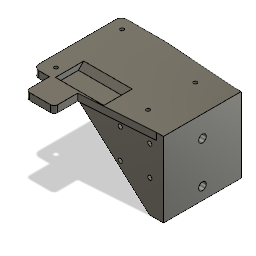
RPLIDAR Bracket v5 (Autodesk Fusion 360 design; units mm, degrees)
Autodesk Fusion 360 part; units mm, degrees
note: some values were not read from the file. Set by a fixed rule: which sketch regions a step uses.
sketch "Sketch1" plane through (0, 0, 0) normal (0, 1, 0) x (1, 0, 0)
  line L0 (0, 0) -> (-5, 0) construction
  line L1 (-5, 0) -> (-33.0162, 0) construction
  line L2 (0, 0) -> (0, 35) construction
  circle A0 centre (-28, 28) radius 1.5
  circle A1 centre (42, 20) radius 1.5
  circle A2 centre (-28, -28) radius 1.5
  circle A3 centre (42, -20) radius 1.5
  line L3 (-38, 0) -> (-38, 37.5)
  line L4 (-38, 37.5) -> (0, 37.5)
  line L5 (0, 37.5) -> (62, 33)
  line L6 (62, 33) -> (62, 0)
  line L7 (62, -33) -> (62, 0)
  line L8 (0, -37.5) -> (62, -33)
  line L9 (-38, -37.5) -> (0, -37.5)
  line L10 (-38, 0) -> (-38, -37.5)
  dimension "d1" = 3
  dimension "d2" = 3
  dimension "d3" = 40
  dimension "d4" = 56
  dimension "d5" = 70
  dimension "d6" = 42
  dimension "d7" = 75
  dimension "d8" = 100
  dimension "d9" = 10
  dimension "d10" = 33
  constraint coincident L0.start L2.start
  constraint horizontal L0
  constraint parallel L0 L1
  constraint perpendicular L0 L2
  constraint symmetric L1 A0 A2
  constraint symmetric L1 A1 A3
  constraint perpendicular L2 L4
  constraint parallel L2 L6
  constraint symmetric L1 L3.start L10.start
  constraint symmetric L1 L3.end L9.start
  constraint symmetric L1 L4.end L8.start
  constraint symmetric L1 L5.end L7.start
  constraint symmetric L1 L6.end L7.end
  constraint vertical L3
  constraint coincident L2 L4.end
  constraint coincident L6.end L7.end
  constraint coincident L3.start L10.start
  measures "d1" diameter of A0
  measures "d2" diameter of A1
  measures "d3" distance of A1.centre A3.centre
  measures "d4" distance of A0.centre A2.centre
  measures "d5" horizontal distance of A0.centre A1.centre
  measures "d6" horizontal distance of L0.start A1.centre
  measures "d7" distance of L3.end L9.start
  measures "d8" distance of L3 L6
  measures "d9" distance of A0.centre L3
  measures "d10" distance of L5.end L6.end
  measures "d20" angle of L4.end
extrude "Extrude1" add sketch "Sketch1" along normal blind 6
ref_plane "WorkPlane1" through (0, 0, 27) normal (0, 0, 1) x (1, 0, 0)
sketch "Sketch3" plane through (0, 0, 27) normal (0, 0, 1) x (1, 0, 0)
  line L0 (-8, 0) -> (62, 0)
  line L1 (62, -57.6259) -> (56, -57.6259)
  line L2 (56, -57.6259) -> (-8, 0)
  line L3 (62, 0) -> (62, -57.6259)
  line L4 (54.1896, -11.7055) -> (54.187, -11.7094)
  point P0 (5, 0)
  dimension "d19" = 6
  dimension "d20" = 42
  dimension "d21" = 70
  constraint vertical L3
  constraint perpendicular L0 L3
  constraint coincident L0.end L4
  constraint perpendicular L1 L3
  constraint coincident P0 L0
  constraint coincident origin L0
  measures "d19" distance of L1.end L1.start
  measures "d20" angle of L0 L2
  measures "d21" distance of L0.start L0.end
extrude "Extrude3" add sketch "Sketch3" along normal blind 6
mirror "Mirror1" about plane through (0, 0, 0) normal (0, 0, 1) of "Extrude3"
sketch "Sketch4" plane through (62, 0, 0) normal (1, 0, 0) x (0, 0, -1)
  line L0 (-27, 0) -> (27, 0)
  line L1 (27, 0) -> (27, -57.6259)
  line L2 (27, -57.6259) -> (33, -57.6259)
  line L3 (33, -57.6259) -> (33, 0)
  line L4 (-33, 0) -> (-33, -57.6259)
  line L5 (-33, -57.6259) -> (-27, -57.6259)
  line L6 (-27, -57.6259) -> (-27, 0)
  line L7 (-33, 6) -> (33, 6)
  line L8 (33, 6) -> (33, -57.6259)
  line L9 (33, -57.6259) -> (-33, -57.6259)
  line L10 (-33, -57.6259) -> (-33, 6)
  circle A0 centre (0, -12) radius 3.25
  circle A1 centre (0, -47) radius 3.25
  line L11 (33, 0) -> (33, 6)
  line L12 (33, 6) -> (-33, 6)
  line L13 (-33, 6) -> (-33, 0)
  dimension "d27" = 6.5
  dimension "d28" = 6.5
  dimension "d29" = 35
  dimension "d30" = 12
  constraint horizontal L7
  constraint vertical L8
  constraint horizontal L9
  constraint vertical L10
  constraint coincident L2.end L3.start
  measures "d27" diameter of A1
  measures "d28" diameter of A0
  measures "d29" distance of A0.centre A1.centre
  measures "d30" distance of L0 A0.centre
extrude "Extrude4" add sketch "Sketch4" along normal blind 6
fillet "Fillet1" radius 5 2 edges at (-38, 3, 37.5) (-38, 3, -37.5)
sketch "Sketch5" plane through (0, 6, 0) normal (0, 1, 0) x (-1, 0, 0)
  arc A0 (33, -37.5) -> (38, -32.5) centre (33, -32.5) ccw
  line L0 (38, -32.5) -> (38, 32.5)
  arc A1 (38, 32.5) -> (33, 37.5) centre (33, 32.5) ccw
  line L1 (33, 37.5) -> (0, 37.5)
  line L2 (0, 37.5) -> (-62, 33)
  line L3 (-62, 33) -> (-68, 33)
  line L4 (0, -37.5) -> (33, -37.5)
  circle A2 centre (28, 28) radius 1.5
  circle A3 centre (-42, 20) radius 1.5
  circle A4 centre (28, -28) radius 1.5
  line L5 (24, 37.5) -> (24, 57.5)
  line L6 (24, 57.5) -> (0, 57.5)
  line L7 (0, 57.5) -> (0, 37.5)
  line L8 (0, 37.5) -> (24, 37.5)
  dimension "d32" = 20
  dimension "d33" = 24
  constraint coincident L1 L5.start
  constraint perpendicular L1 L5
  constraint coincident L1.end L2.start
  constraint perpendicular L1 L7
  constraint horizontal L6
  measures "d32" distance of L5.start L5.end
  measures "d33" distance of L5.end L6.end
extrude "Extrude5" add sketch "Sketch5" against normal blind 6 contours L1 L5 L6 L7 L8
fillet "Fillet2" radius 3 2 edges at (-24, 3, 57.5) (0, 3, 57.5)
sketch "Sketch6" plane through (0, 6, 0) normal (0, 1, 0) x (-1, 0, 0)
  arc A0 (3, 57.5) -> (0, 54.5) centre (3, 54.5) ccw
  line L0 (0, 54.5) -> (0, 37.5)
  line L1 (0, 37.5) -> (-62, 33)
  line L2 (-62, 33) -> (-68, 33)
  line L3 (-68, 33) -> (-68, -33)
  line L4 (-68, -33) -> (-62, -33)
  line L5 (-62, -33) -> (0, -37.5)
  line L6 (0, -37.5) -> (33, -37.5)
  arc A1 (33, -37.5) -> (38, -32.5) centre (33, -32.5) ccw
  line L7 (38, -32.5) -> (38, 32.5)
  arc A2 (38, 32.5) -> (33, 37.5) centre (33, 32.5) ccw
  line L8 (33, 37.5) -> (24, 37.5)
  line L9 (24, 37.5) -> (24, 54.5)
  arc A3 (24, 54.5) -> (21, 57.5) centre (21, 54.5) ccw
  line L10 (21, 57.5) -> (3, 57.5)
  circle A4 centre (28, 28) radius 1.5
  circle A5 centre (-42, 20) radius 1.5
  circle A6 centre (-42, -20) radius 1.5
  circle A7 centre (28, -28) radius 1.5
  line L11 (21, 16) -> (-20, 16)
  line L12 (-20, 16) -> (-20, 30.9726)
  line L13 (-20, 30.9726) -> (21, 30.9726)
  line L14 (21, 30.9726) -> (21, 16)
  constraint horizontal L11
  constraint vertical L12
  constraint horizontal L13
  constraint vertical L14
extrude "Extrude6" cut sketch "Sketch6" against normal blind 4.5 contours L11 L12 L13 L14
chamfer "Chamfer1" distance 4.5 angle 45 2 edges at (-0.5, 6, 30.9726) (-0.5, 6, 16)
sketch "Sketch7" plane through (0, 0, 33) normal (0, 0, 1) x (1, 0, 0)
  line L0 (62, 0) -> (-8, 0)
  line L1 (-8, 0) -> (56, -57.6259) construction
  line L2 (56, -57.6259) -> (68, -57.6259)
  line L3 (68, -57.6259) -> (68, 6) construction
  line L4 (68, 6) -> (62, 6)
  line L5 (62, 6) -> (62, 0)
  line L6 (56.4712, -5.0375) -> (31.4712, -5.0375) construction
  line L7 (31.4712, -5.0375) -> (31.4712, -30.0375) construction
  line L8 (31.4712, -30.0375) -> (56.4712, -30.0375) construction
  line L9 (56.4712, -30.0375) -> (56.4712, -5.0375) construction
  line L10 (56.4712, -5.0375) -> (31.4712, -30.0375) construction
  line L11 (31.4712, -5.0375) -> (56.4712, -30.0375) construction
  circle A0 centre (56.4712, -5.0375) radius 1.75
  line L12 (43.9712, -17.5375) -> (43.9712, -12) construction
  line L13 (43.9712, -17.5375) -> (51.6365, -17.5375) construction
  circle A1 centre (31.4712, -5.0375) radius 1.75
  circle A2 centre (31.4712, -30.0375) radius 1.75
  circle A3 centre (56.4712, -30.0375) radius 1.75
  point P0 (43.9712, -17.5375)
  dimension "d43" = 25
  dimension "d44" = 25
  dimension "d45" = 3.5
  constraint perpendicular L6 L7
  constraint parallel L6 L8
  constraint parallel L7 L9
  constraint horizontal L6
  constraint coincident L10 P0
  constraint coincident L11 P0
  constraint coincident L6.start L9.end
  constraint coincident P0 L12.start
  constraint perpendicular L8 L12
  constraint perpendicular L12 L13
  constraint symmetric A0 L12 A1
  constraint symmetric A0 L13 A3
  constraint symmetric L13 A1 A2
  measures "d43" distance of L6.start L8.end
  measures "d44" distance of L6.start L6.end
  measures "d45" diameter of A0
extrude "Extrude7" cut sketch "Sketch7" against normal up to surface (6 mm away)
equation "d5 = 28 mm + 42 mm"
